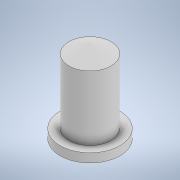
# Autodesk Inventor part: PuntaMarcador
Saved by Autodesk Inventor 2022 (Build 260153000, 153)
## iProperties
Created: 2022-08-28
Part Number: PuntaMarcador
Material: Generic
Document SubType Name: Modeling
Designer: Usuario
Density: 1 g/cm^3
Appearance: Default
Author: Usuario
Autodesk Inventor part; units mm, degrees
ref_plane "YZ Plane" through (0, 0, 0) normal (1, 0, 0) x (0, 1, 0)
ref_plane "XZ Plane" through (0, 0, 0) normal (0, 1, 0) x (-1, 0, 0)
ref_plane "XY Plane" through (0, 0, 0) normal (0, 0, 1) x (1, 0, 0)
sketch "Sketch1" plane through (0, 0, 0) normal (0, 0, 1) x (1, 0, 0)
  line L0 (4.75, 16.5798) -> (4.75, 2)
  line L1 (4.75, 2) -> (6.75, 2)
  line L2 (6.75, 2) -> (6.75, 0)
  line L3 (6.75, 0) -> (0, 0)
  line L4 (0, 20.9758) -> (0, -3.9256)
  line L5 (0, 19) -> (4.75, 16.5798)
  dimension "d0" = 2
  dimension "d1" = 2
  dimension "d3" = 9.5
  dimension "d5" = 117
  dimension "d6" = 19
  constraints: 12 end point, 3 perpendicular, 2 point on line, 1 vertical
  measures "d0" distance of L1.end L2.end
  measures "d1" distance of L0.end L1.end
  measures "d3" diameter of L0 L4
  measures "d5" angle of L0 L5
  measures "d6" distance from line of L5.start L3
revolve "Revolution1" add sketch "Sketch1" angle 360 about axis through (0, 20.9758, 0) along (0, -1, 0)
body "Solid1"
